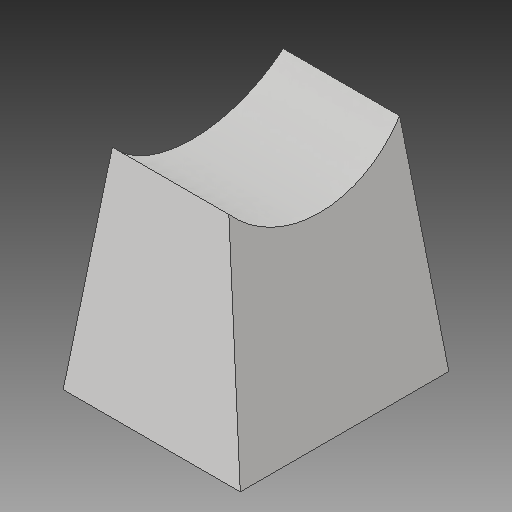
# Autodesk Inventor part: BaseGarra
Saved by Autodesk Inventor 2019 (Build 230136000, 136)
## iProperties
Created: 2020-01-20
Part Number: BaseGarra
Material: Generic
Document SubType Name: Modeling
Designer: peter
Density: 1 g/cm^3
Appearance: Default
Author: peter
Autodesk Inventor part; units mm, degrees
ref_plane "YZ Plane" through (0, 0, 0) normal (1, 0, 0) x (0, 1, 0)
ref_plane "XZ Plane" through (0, 0, 0) normal (0, 1, 0) x (-1, 0, 0)
ref_plane "XY Plane" through (0, 0, 0) normal (0, 0, 1) x (1, 0, 0)
sketch "Sketch1" plane through (0, 0, 0) normal (1, 0, 0) x (0, 1, 0)
  arc A0 (-3.4223, -4.604) -> (-3.4223, -18.104) centre (2.5306, -11.354) ccw
  line L0 (-20.4694, -3.1126) -> (-20.4694, -19.5954)
  line L1 (-3.4223, -18.104) -> (-20.4694, -19.5954)
  line L2 (-3.4223, -4.604) -> (-20.4694, -3.1126)
  point P0 (0, 0)
  dimension "d5" = 23
  dimension "d21" = 9
  dimension "d28" = 85
  constraints: 6 end point, 2 point on circle, 1 centre point, 1 vertical
  measures "d5" distance from line of L0 A0.centre
  measures "d21" radius of A0
  measures "d28" angle of L0 L1
extrude "Extrusion1" add sketch "Sketch1" along normal blind 14
draft "FaceDraft3" angle 8 pull direction (0, 1, 0) faces at (0, -15.7807, -10.9914) fixed edges at (0, -20.4694, -11.354)
draft "FaceDraft4" angle 8 pull direction (0, 1, 0) faces at (14, -15.7807, -10.9914) fixed edges at (14, -20.4694, -11.354)
body "Solid1"
